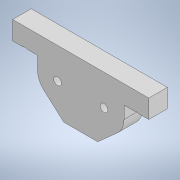
# Autodesk Inventor part: ベルト固定_アルミ
Saved by Autodesk Inventor 2021 (Build 250183000, 183)
## iProperties
Created: 2022-02-24
Part Number: ベルト固定_アルミ
Material: 一般
Document SubType Name: Modeling
Designer: hirohumi
Density: 1 g/cm^3
Appearance: 既定
Author: hirohumi
Autodesk Inventor part; units mm, degrees
ref_plane "YZ Plane" through (0, 0, 0) normal (1, 0, 0) x (0, 1, 0)
ref_plane "XZ Plane" through (0, 0, 0) normal (0, 1, 0) x (-1, 0, 0)
ref_plane "XY Plane" through (0, 0, 0) normal (0, 0, 1) x (1, 0, 0)
sketch "スケッチ1" plane through (0, 0, 0) normal (0, 0, 1) x (1, 0, 0)
  circle A0 centre (-7.5, 0) radius 1.25
  circle A1 centre (7.5, 0) radius 1.25
  line L0 (-14, -10.5) -> (-5.5, -10.5) construction
  line L1 (22, 10) -> (-22, 10)
  arc A2 (-18.7483, 4) -> (-17.2517, 4) centre (-18, 2.7) ccw construction
  arc A3 (17.2517, 4) -> (18.7483, 4) centre (18, 2.7) ccw construction
  line L2 (-22, 10) -> (-22, 4)
  line L3 (-22, 4) -> (-18.7483, 4)
  line L4 (-14, 4) -> (-14, 0)
  line L5 (22, 10) -> (22, 4)
  line L6 (22, 4) -> (18.7483, 4)
  line L7 (14, 4) -> (14, 0)
  arc A4 (-17.2517, 4) -> (-18.7483, 4) centre (-18, 2.7) ccw
  line L8 (-18.7483, 4) -> (-17.2517, 4) construction
  line L9 (-17.2517, 4) -> (-14, 4)
  arc A5 (18.7483, 4) -> (17.2517, 4) centre (18, 2.7) ccw
  line L10 (18.7483, 4) -> (17.2517, 4) construction
  line L11 (17.2517, 4) -> (14, 4)
  arc A6 (-14, 0) -> (-11.8293, -4.8484) centre (-7.5, 0) ccw
  arc A7 (11.8293, -4.8484) -> (14, 0) centre (7.5, 0) ccw
  line L12 (-11.8293, -4.8484) -> (-5.5, -10.5)
  line L13 (11.8293, -4.8484) -> (5.5, -10.5)
  line L14 (-14, 0) -> (-14, -10.5) construction
  line L15 (-5.5, -10.5) -> (5.5, -10.5)
  line L16 (5.5, -10.5) -> (14, -10.5) construction
  line L17 (14, 0) -> (14, -10.5) construction
  point P0 (0, 0)
  dimension "d0" = 2.5
  dimension "d1" = 2.5
  dimension "d2" = 15
  dimension "d3" = 7.5
  dimension "d8" = 10.5
  dimension "d9" = 10
  dimension "d15" = 3
  dimension "d16" = 3
  dimension "d21" = 6.5
  dimension "d22" = 6.5
  dimension "d23" = 10.5
  dimension "d24" = 6
  dimension "d25" = 6
  dimension "d26" = 8
  dimension "d27" = 8
  dimension "d28" = 1.3
  dimension "d29" = 1.3
  dimension "d30" = 4
  dimension "d31" = 4
  dimension "d34" = 11
  dimension "d35" = 5.5
  constraints: 36 end point, 12 point on circle, 8 centre point, 6 perpendicular, 6 tangent, 6 vertical, 3 point on line, 2 coincident, 2 horizontal alignment, 1 horizontal
  measures "d0" diameter of A0
  measures "d1" diameter of A1
  measures "d2" distance of A1.centre A0.centre
  measures "d3" distance of point (0, 0) A0.centre
  measures "d8" distance from line of L0 A0.centre
  measures "d9" distance from line of L1 A0.centre
  measures "d15" diameter of A2
  measures "d16" diameter of A3
  measures "d21" distance from line of A0.centre L4
  measures "d22" distance from line of L7 A1.centre
  measures "d23" distance from line of L0 A1.centre
  measures "d24" distance between parallel lines of L3 L1
  measures "d25" distance between parallel lines of L6 L1
  measures "d26" distance between parallel lines of L4 L2
  measures "d27" distance between parallel lines of L7 L5
  measures "d28" distance from line of L3 A2.centre
  measures "d29" distance from line of L6 A3.centre
  measures "d30" distance from line of A3.centre L5
  measures "d31" distance from line of A2.centre L2
  measures "d34" distance of L13.end L0.end
  measures "d35" horizontal distance of point (0, 0) L0.end
extrude "押し出し1" add sketch "スケッチ1" along normal blind 6
equation "\"d3\" = 0.5 * d2"
equation "\"d35\" = 0.5 * d34"
